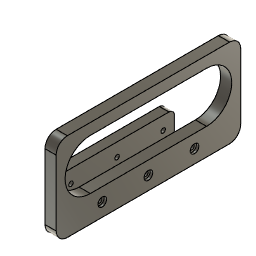
laundry-handle (Autodesk Fusion 360 design; units mm, degrees)
Autodesk Fusion 360 part; units mm, degrees
sketch "Sketch1" plane through (0, 0, 0) normal (1, 0, 0) x (0, 1, 0)
  line L0 (0, 0) -> (165, 0)
  circle A0 centre (41.25, 11.875) radius 3.875
  circle A1 centre (41.25, 11.875) radius 2
  line L1 (0, 0) -> (0, 78.75)
  line L2 (0, 78.75) -> (165, 78.75)
  line L3 (165, 78.75) -> (165, 0)
  line L4 (-0.2625, 46.25) -> (164.7378, 46.25) construction
  line L5 (30.5, 23.75) -> (134.5, 23.75)
  arc A2 (134.5, 23.75) -> (134.5, 68.75) centre (134.5, 46.25) ccw
  line L6 (134.5, 68.75) -> (30.5, 68.75)
  arc A3 (30.5, 68.75) -> (30.5, 23.75) centre (30.5, 46.25) ccw
  line L7 (30.5, 46.25) -> (134.5, 46.25) construction
  line L8 (82.5, 0) -> (82.5, 23.75) construction
  line L9 (82.5, 11.875) -> (0, 11.875) construction
  line L10 (41.25, 11.875) -> (41.25, 0) construction
  circle A4 centre (123.75, 11.875) radius 3.875
  circle A5 centre (123.75, 11.875) radius 2
  circle A6 centre (82.5, 11.875) radius 2
  circle A7 centre (82.5, 11.875) radius 3.875
  dimension "d1" = 165
  dimension "d3" = 7.75
  dimension "d4" = 4
  dimension "d8" = 45
  dimension "d13" = 10
  dimension "d14" = 8
  dimension "d15" = 8
  dimension "d16" = 8
  dimension "d17" = 8
  dimension "d35" = 4
  dimension "d36" = 7.75
  constraint horizontal L0
  constraint coincident L0.start L1.start
  constraint concentric A0 A1
  constraint tangent L5 A2
  constraint tangent A2 L6
  constraint parallel L5 L6
  constraint tangent L6 A3
  constraint tangent L5 A3
  constraint coincident L4 A2.centre
  constraint parallel L4 L7
  constraint midpoint L0 L8.start
  constraint midpoint L5 L8.end
  constraint perpendicular L2 L3
  constraint perpendicular L1 L2
  constraint perpendicular L0 L1
  constraint midpoint L8 L9.start
  constraint coincident L1 L9.end
  constraint perpendicular L1 L9
  constraint midpoint L9 A0.centre
  constraint coincident L0 L10.end
  constraint perpendicular L0 L10
  constraint coincident A0.centre A1.centre
  constraint symmetric A0 L8 A4
  constraint symmetric A1 L8 A5
  constraint coincident L9.start A6.centre
  constraint concentric A6 A7
  measures "d1" distance of L0.start L0.end
  measures "d3" diameter of A0
  measures "d4" diameter of A1
  measures "d8" distance of L5 L6
  measures "d13" distance of L2 L6
  measures "d14" distance of L0 A0
  measures "d15" distance of A0 L5
  measures "d16" distance of L1 A3
  measures "d17" distance of L3 A2
  measures "d35" diameter of A6
  measures "d36" diameter of A7
extrude "Extrude1" add sketch "Sketch1" along normal blind 10 contours L0 L1 L2 L3 | A0 | A4 | A7 makes body 1
extrude "Extrude2" cut sketch "Sketch1" against normal blind 2.25 from surface at 10 contours A0 | A4 | A7 bodies 1
sketch "Sketch2" plane through (0, 0, 0) normal (-1, 0, 0) x (0, -1, 0)
  circle A0 centre (-41.25, 11.875) radius 2
  arc A1 (-134.5, 68.75) -> (-134.5, 23.75) centre (-134.5, 46.25) ccw
  line L0 (-134.5, 23.75) -> (-30.5, 23.75)
  line L1 (0, 0) -> (-165, 0)
  line L2 (-165, 78.75) -> (-165, 0)
  line L3 (0, 78.75) -> (-165, 78.75)
  line L4 (-30.5, 68.75) -> (-134.5, 68.75)
  arc A2 (-30.5, 23.75) -> (-30.5, 68.75) centre (-30.5, 46.25) ccw
  line L5 (0, 0) -> (0, 78.75)
  circle A3 centre (-123.75, 11.875) radius 2
  line L6 (-82.5, 78.75) -> (-82.5, 0) construction
  line L7 (-134.5, 23.75) -> (-165, 23.75)
  line L8 (-30.5, 23.75) -> (0, 23.75)
  line L9 (-133.75, 23.75) -> (-133.75, 0)
  line L10 (-120.25, 13.8957) -> (-123.75, 15.9165)
  line L11 (-123.75, 15.9165) -> (-127.25, 13.8957)
  line L12 (-127.25, 13.8957) -> (-127.25, 9.8543)
  line L13 (-127.25, 9.8543) -> (-123.75, 7.8335)
  line L14 (-123.75, 7.8335) -> (-120.25, 9.8543)
  line L15 (-120.25, 9.8543) -> (-120.25, 13.8957)
  line L16 (-44.75, 13.8957) -> (-41.25, 15.9165)
  line L17 (-44.75, 9.8543) -> (-44.75, 13.8957)
  line L18 (-41.25, 7.8335) -> (-44.75, 9.8543)
  line L19 (-37.75, 9.8543) -> (-41.25, 7.8335)
  line L20 (-37.75, 13.8957) -> (-37.75, 9.8543)
  line L21 (-41.25, 15.9165) -> (-37.75, 13.8957)
  line L22 (-31.25, 23.75) -> (-31.25, 0)
  circle A4 centre (-82.5, 11.875) radius 2
  line L23 (-82.5, 7.8335) -> (-79, 9.8543)
  line L24 (-79, 9.8543) -> (-79, 13.8957)
  line L25 (-79, 13.8957) -> (-82.5, 15.9165)
  line L26 (-82.5, 15.9165) -> (-86, 13.8957)
  line L27 (-86, 13.8957) -> (-86, 9.8543)
  line L28 (-86, 9.8543) -> (-82.5, 7.8335)
  point P0 (-123.75, 11.875)
  point P1 (-82.5, 11.875)
  dimension "d23" = 8
  dimension "d25" = 7
  dimension "d37" = 7
  constraint midpoint L3 L6.start
  constraint midpoint L1 L6.end
  constraint coincident A1.end L0.start
  constraint coincident L2 L7.end
  constraint tangent A1 L7
  constraint coincident L0.end A2.start
  constraint coincident L5 L8.end
  constraint tangent A2 L8
  constraint coincident L7 L9.start
  constraint coincident L1 L9.end
  constraint perpendicular L1 L9
  constraint coincident P0 A3.centre
  constraint parallel L9 L12
  constraint symmetric L6 L9.start L22.start
  constraint symmetric L6 L9.end L22.end
  constraint symmetric L6 L10.start L16.start
  constraint symmetric L6 L10.end L16.end
  constraint symmetric L6 L11.end L20.start
  constraint symmetric L6 L12.end L19.start
  constraint symmetric L6 L13.end L18.start
  constraint symmetric L6 L14.end L17.start
  constraint coincident P1 A4.centre
  constraint parallel L15 L27
  measures "d23" distance of A3 L9
  measures "d25" distance of L12 L15
  measures "d37" distance of L25 L28
extrude "Extrude3" add sketch "Sketch2" along normal blind 8.5 separate body contours L0 L1 L9 L22 | L10 L11 L12 L13 L14 L15 | L16 L17 L18 L19 L20 L21 | L23 L24 L25 L26 L27 L28 makes body 2
extrude "Extrude4" cut sketch "Sketch2" against normal blind 3.25 from surface at 8.5 contours L10 L11 L12 L13 L14 L15 | L16 L17 L18 L19 L20 L21 | L23 L24 L25 L26 L27 L28 bodies 2
move_body "Move1" bodies 2 to x (1, 0, 0) y (0, 1, 0) z (0, 0, 1) at (-18, 0, 0)
fillet "Fillet1" radius 5 4 edges at (-22.25, 133.75, 23.75) (-22.25, 133.75, 0) (-22.25, 31.25, 23.75) (-22.25, 31.25, 0) on bodies 2
fillet "Fillet2" radius 10 4 edges at (5, 165, 78.75) (5, 165, 0) (5, 0, 78.75) (5, 0, 0) on bodies 1
named bodies: "laundry-handle-front", "laundry-handle-back"
